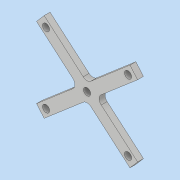
# Autodesk Inventor part: cellSTORM_inverted_LED
Saved by Autodesk Inventor 2019.4 (Build 234330000, 330)
## iProperties
Created: 2020-12-11
Part Number: cellSTORM_inverted_LED
Material: Generic
Document SubType Name: Modeling
Designer: diederichbenedict
Density: 1 g/cm^3
Appearance: Default
Author: diederichbenedict
Autodesk Inventor part; units mm, degrees
ref_plane "YZ Plane" through (0, 0, 0) normal (1, 0, 0) x (0, 1, 0)
ref_plane "XZ Plane" through (0, 0, 0) normal (0, 1, 0) x (-1, 0, 0)
ref_plane "XY Plane" through (0, 0, 0) normal (0, 0, 1) x (1, 0, 0)
sketch "Sketch1" plane through (0, 0, 0) normal (0, 0, 1) x (1, 0, 0)
  circle A0 centre (0, 0) radius 3 projected
  circle A1 centre (0, -60) radius 3 projected
  circle A2 centre (70, 0) radius 3 projected
  circle A3 centre (70, -60) radius 3.05 projected
  circle A4 centre (37.1599, -42) radius 6.15 construction
  line L0 (70, 0) -> (0, -60) construction
  line L1 (70, -60) -> (0, 0) construction
  circle A5 centre (35, -30) radius 2.5 construction
  line L2 (-1.607, 7.9628) -> (78.1149, -60.3703)
  line L3 (78.1149, -60.3703) -> (71.607, -67.9628)
  line L4 (71.607, -67.9628) -> (-8.1149, 0.3703)
  line L5 (-8.1149, 0.3703) -> (-1.607, 7.9628)
  line L6 (-1.607, 7.9628) -> (71.607, -67.9628) construction
  line L7 (78.1149, -60.3703) -> (-8.1149, 0.3703) construction
  line L8 (78.1149, 0.3703) -> (-1.607, -67.9628)
  line L9 (-1.607, -67.9628) -> (-8.1149, -60.3703)
  line L10 (-8.1149, -60.3703) -> (71.607, 7.9628)
  line L11 (71.607, 7.9628) -> (78.1149, 0.3703)
  line L12 (78.1149, 0.3703) -> (-8.1149, -60.3703) construction
  line L13 (-1.607, -67.9628) -> (71.607, 7.9628) construction
  point P0 (0, 0)
  dimension "d0" = 5
  dimension "d1" = 105
  dimension "d2" = 10
  dimension "d3" = 105
  dimension "d4" = 10
  constraints: 28 end point, 5 midpoint, 4 parallel, 2 perpendicular, 1 centre point, 1 coincident
  measures "d0" diameter of A5
  measures "d1" distance of L2.start L2.end
  measures "d2" distance of L2.end L3.end
  measures "d3" distance of L8.start L8.end
  measures "d4" distance of L8.end L9.end
extrude "Extrusion1" add sketch "Sketch1" along normal blind 5
sketch "Sketch2" plane through (0, 0, 5) normal (0, 0, 1) x (1, 0, 0)
  circle A0 centre (0, -60) radius 3 projected
  circle A1 centre (70, 0) radius 3 projected
  circle A2 centre (70, -60) radius 3.05 projected
  circle A3 centre (0, 0) radius 3 projected
  line L0 (35, -23.4146) -> (-1.607, 7.9628) projected
  line L1 (-1.607, 7.9628) -> (-8.1149, 0.3703) projected
  line L2 (-8.1149, 0.3703) -> (27.317, -30) projected
  line L3 (27.317, -30) -> (-8.1149, -60.3703) projected
  line L4 (-8.1149, -60.3703) -> (-1.607, -67.9628) projected
  line L5 (-1.607, -67.9628) -> (35, -36.5854) projected
  line L6 (35, -36.5854) -> (71.607, -67.9628) projected
  line L7 (71.607, -67.9628) -> (78.1149, -60.3703) projected
  line L8 (78.1149, -60.3703) -> (42.683, -30) projected
  line L9 (42.683, -30) -> (78.1149, 0.3703) projected
  line L10 (78.1149, 0.3703) -> (71.607, 7.9628) projected
  line L11 (71.607, 7.9628) -> (35, -23.4146) projected
  circle A4 centre (35, -30) radius 3
  point P0 (0, 0)
  dimension "d7" = 6
  constraints: 1 centre point
  measures "d7" diameter of A4
extrude "Extrusion2" cut sketch "Sketch2" against normal through all contours A4
fillet "Fillet1" radius 5 4 edges at (35, -23.4146, 2.5) (27.317, -30, 2.5) (35, -36.5854, 2.5) (42.683, -30, 2.5)
body "Solid1"
